Autodesk Inventor part; units mm, degrees
(part 2 of 2)
  circle A352 centre (1.9365, 27.8521) radius 31.0271
  dimension "d26" = 55.7042
  dimension "d27" = 3.175
  constraints: 3 coincident, 2 centre point, 3 other
  measures "d26" diameter of A350
  measures "d27" radial gap between concentric circles of A350 A352
extrude "Extrusion2" add sketch "Sketch3" against normal up to surface (9 mm away) contours A350
extrude "Extrusion3" cut sketch "Sketch3" against normal up to surface (9 mm away) contours A352
body "Solid1"
